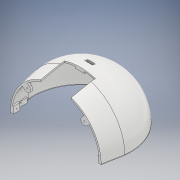
# Autodesk Inventor part: back
Saved by Autodesk Inventor 2017 (Build 210142000, 142)
## iProperties
Part Number: back
Material: Genérico
Document SubType Name: Modeling
Designer: Roberto
Density: 1 g/cm^3
Appearance: Valor por defecto
Author: Roberto
Autodesk Inventor part; units mm, degrees
ref_plane "YZ Plane" through (0, 0, 0) normal (1, 0, 0) x (0, 1, 0)
ref_plane "XY Plane" through (0, 0, 0) normal (0, 0, 1) x (1, 0, 0)
sketch "Boceto1" plane through (0, 0, 0) normal (0, 0, 1) x (1, 0, 0)
  line L0 (0, 0) -> (0.3056, 0)
  line L1 (-0.374, 3.3479) -> (0.2767, 0)
  line L2 (-0.6113, 3.2908) -> (0, 0)
  arc A0 (3.9618, 11.347) -> (-0.374, 3.3479) centre (7.6858, 4.1538) ccw
  arc A1 (3.8504, 11.5616) -> (-0.6113, 3.2908) centre (7.6858, 4.1538) ccw
  line L3 (0, 0) -> (15, 0)
  arc A2 (7.5, 12.385) -> (3.8946, 11.3118) centre (8.3964, 2.7813) ccw
  arc A3 (7.5, 12.6279) -> (3.8504, 11.5616) centre (8.3964, 2.7813) ccw
  line L4 (0, 0) -> (0.3056, 0)
  line L5 (0.2767, 0) -> (-0.374, 3.3479)
  line L6 (-0.6113, 3.2908) -> (0, 0)
  line L7 (-0.6113, 3.2908) -> (-0.374, 3.3479)
  line L8 (0.2767, 0) -> (0, 0)
  line L9 (7.5, 12.6279) -> (7.5, 12.385)
  dimension "d0" = 15
  constraints: 20 end point, 11 point on circle, 4 centre point, 3 collinear, 3 horizontal, 2 coincident, 1 vertical
  measures "d0" distance of L0.start L3.end
revolve "Revolución1" add sketch "Boceto1" angle 180 about axis through (7.5, 12.6279, 0) along (0, 1, 0)
sketch "Boceto2" plane through (7.5, 0, 0) normal (0, -1, 0) x (1, 0, 0)
  circle A0 centre (4.734, 4.734) radius 0.1
  circle A1 centre (-4.734, 4.734) radius 0.1
  arc A2 (7.5, 0) -> (-7.5, 0) centre (0, 0) ccw projected
  arc A3 (-5.1946, 4.3495) -> (-4.3495, 5.1946) centre (-4.734, 4.734) ccw
  line L0 (-4.2734, 5.1185) -> (-4.7635, 5.6086)
  line L1 (-5.1185, 4.2734) -> (-5.6117, 4.7666)
  line L2 (0, 0) -> (0, 11.2939)
  circle A4 centre (4.734, 4.734) radius 0.1
  arc A5 (7.5, 0) -> (-7.5, 0) centre (0, 0) ccw
  arc A6 (4.3495, 5.1946) -> (5.1946, 4.3495) centre (4.734, 4.734) ccw
  line L3 (4.2734, 5.1185) -> (4.8639, 5.709)
  line L4 (5.1185, 4.2734) -> (5.6108, 4.7657)
  line L5 (-4.6631, 5.5082) -> (-4.7635, 5.6086)
  line L6 (-5.5144, 4.6693) -> (-5.6117, 4.7666)
  line L7 (-5.6117, 4.7666) -> (-4.7635, 5.6086)
  arc A7 (7.2233, 0) -> (-7.2233, 0) centre (0, 0) ccw projected
  line L8 (5.5127, 4.6675) -> (5.6108, 4.7657)
  line L9 (4.6675, 5.5127) -> (4.7657, 5.6108)
  line L10 (4.7657, 5.6108) -> (5.6108, 4.7657)
  point P0 (-4.8639, 5.709)
  point P1 (-5.709, 4.8639)
  point P2 (5.709, 4.8639)
  dimension "d2" = 1.2
  dimension "d109" = 0.2
  dimension "d110" = 0.2
  constraints: 22 end point, 12 point on circle, 10 symmetric about line, 8 point on line, 6 centre point, 2 coincident, 2 parallel, 1 collinear, 1 vertical, 3 other
  measures "d2" diameter of A3
  measures "d109" diameter of A0
  measures "d110" diameter of A1
extrude "Extrusión1" add sketch "Boceto2" against normal blind 0.3 contours L10 L4 A7 L3 | A7 L4 A6 L3 | L1 A7 L0 A3 | L1 L7 L0 A7
sketch "Boceto4" plane through (7.6858, 4.1538, 0) normal (0, 0, -1) x (-0.8801071, 0.4747751, 0)
  line L0 (2.2994, -5.96) -> (-5.9165, -1.5279) projected
  line L1 (-4.0528, -2.5333) -> (-2.1537, 0.9871)
  line L2 (-2.1537, 0.9871) -> (2.3348, -1.4342)
  line L3 (2.3348, -1.4342) -> (0.4357, -4.9546)
  line L4 (-4.0528, -2.5333) -> (0.4357, -4.9546)
  line L5 (4.7922, -7.3048) -> (-8.4094, -0.1832) projected
  dimension "d6" = 4
  dimension "d7" = 5.1
  constraints: 8 end point, 2 point on line, 1 collinear, 1 perpendicular
  measures "d6" distance of L1.start L1.end
  measures "d7" distance of L1.end L2.end
extrude "Extrusión2" cut sketch "Boceto4" against normal blind 10
sketch "Boceto5" plane through (7.6858, 4.1538, 0) normal (0, 0, -1) x (-0.8801071, 0.4747751, 0)
  line L0 (-7.385, 3.0033) -> (-8.4094, -0.1832) projected
  line L1 (-8.4094, -0.1832) -> (-8.1658, -0.3145) projected
  line L2 (-8.1658, -0.3145) -> (-7.149, 2.941) projected
  arc A0 (0.3888, 7.9233) -> (-7.149, 2.941) centre (0.3271, -0.1764) ccw projected
  arc A1 (4.0715, 7.1562) -> (0.3888, 7.9233) centre (0.3008, -1.7218) ccw projected
  arc A2 (6.7351, 4.4998) -> (4.0715, 7.1562) centre (-1.277, -0.8706) ccw projected
  arc A3 (6.7109, -4.5358) -> (6.7351, 4.4998) centre (0, 0) ccw projected
  line L3 (4.5487, -7.1734) -> (6.7109, -4.5358) projected
  line L4 (4.7922, -7.3048) -> (4.5487, -7.1734) projected
  line L5 (6.8926, -4.6988) -> (4.7922, -7.3048) projected
  arc A4 (6.8926, -4.6988) -> (6.8926, 4.6988) centre (0, 0) ccw projected
  arc A5 (6.8926, 4.6988) -> (4.1869, 7.37) centre (-1.277, -0.8706) ccw projected
  arc A6 (4.1869, 7.37) -> (0.4686, 8.1642) centre (0.3008, -1.7218) ccw projected
  arc A7 (0.4686, 8.1642) -> (-7.385, 3.0033) centre (0.3271, -0.1764) ccw projected
extrude "Extrusión3" add sketch "Boceto5" along normal blind 0.1
sketch "Boceto6" plane through (7.5, 4, 0) normal (0, -1, 0) x (1, 0, 0)
  arc A0 (2.55, 7.7457) -> (-2.55, 7.7457) centre (0, 0) ccw projected
  line L0 (-2.55, 7.4906) -> (-2.55, 7.7457) projected
  arc A1 (2.55, 7.4906) -> (-2.55, 7.4906) centre (0, 0) ccw projected
  line L1 (2.55, 7.4906) -> (2.55, 7.7457) projected
  arc A2 (2.55, 7.7457) -> (-2.55, 7.7457) centre (0, 0) ccw projected
  line L2 (0, 8.1546) -> (0, 7.9127)
  line L3 (0, 8.0337) -> (-0.75, 8.0337)
  line L4 (-0.75, 8.0337) -> (-0.75, 7.5837)
  line L5 (-0.75, 7.5837) -> (0.75, 7.5837)
  line L6 (0.75, 7.5837) -> (0.75, 8.0337)
  line L7 (0.75, 8.0337) -> (0, 8.0337)
  point P0 (-7.5, 0)
  dimension "d12" = 0.75
  dimension "d13" = 0.45
  dimension "d14" = 1.5
  constraints: 12 end point, 4 perpendicular, 3 point on circle, 1 horizontal, 1 midpoint, 1 point on line
  measures "d12" distance of L3.start L3.end
  measures "d13" distance of L3.end L4.end
  measures "d14" distance of L4.end L5.end
extrude "Extrusión4" add sketch "Boceto6" against normal blind 1.2 contours L7 L6 A1 L2 | L2 A1 L4 L3 | L6 L5 L4 A1
sketch "Boceto7" plane through (8.25, 4, 7.5837) normal (0, 0, -1) x (-1, 0, 0)
  line L0 (1.5, 0) -> (0, 0) projected
  line L1 (1.5, 0) -> (1.5, 1.2) projected
  line L2 (0, 1.2) -> (1.5, 1.2) projected
  line L3 (0, 0) -> (0, 1.2) projected
  line L4 (0, 1.2) -> (1.5, 1.2) projected
  line L5 (3.3, 0) -> (-1.8, 0) projected
  circle A0 centre (0.65, 0.3) radius 0.075
  circle A1 centre (0.65, 0.9) radius 0.075
  point P0 (8.25, -4)
  dimension "d20" = 0.15
  dimension "d21" = 0.15
  constraints: 2 centre point
  measures "d20" diameter of A0
  measures "d21" diameter of A1
extrude "Extrusión5" cut sketch "Boceto7" against normal blind 0.3 contours A0 | A1
ref_plane "Plano de trabajo1" through (0, 2, 0) normal (0, 1, 0) x (-1, 0, 0)
sketch "Boceto12" plane through (0, 2, 0) normal (0, 1, 0) x (-1, 0, 0)
  line L0 (-15, -0.1) -> (-15.6113, -0.1)
  line L1 (-0.3817, -3.084) -> (-1.27, -4.6226)
  line L2 (-1.27, -4.6226) -> (-1.4865, -4.4976)
  line L3 (-4.541, -6.9018) -> (-3.0024, -6.0135)
  line L4 (-2.8774, -6.23) -> (-3.0024, -6.0135)
  line L5 (-0.3817, -3.084) -> (-0.5982, -2.959)
  line L6 (-6.6117, -7.7066) -> (-8.3883, -7.7066)
  line L7 (-8.3883, -7.7066) -> (-8.3883, -7.4566)
  line L8 (-1.4865, -4.4976) -> (-0.5982, -2.959)
  line L9 (-2.8774, -6.23) -> (-4.416, -7.1183)
  line L10 (-4.416, -7.1183) -> (-4.541, -6.9018)
  line L11 (-8.3883, -7.4566) -> (-6.6117, -7.4566)
  line L12 (-6.6117, -7.7066) -> (-6.6117, -7.4566)
  line L13 (-0.0434, -0.1) -> (0.2066, -0.1)
  line L14 (-7.5, 0) -> (-7.5, -4.1757)
  line L15 (-14.6183, -3.084) -> (-13.73, -4.6226)
  line L16 (-13.73, -4.6226) -> (-13.5135, -4.4976)
  line L17 (-15.2066, -1.0883) -> (-14.9566, -1.0883)
  line L18 (-13.5135, -4.4976) -> (-14.4018, -2.959)
  line L19 (-14.6183, -3.084) -> (-14.4018, -2.959)
  line L20 (-15.2066, -1.0883) -> (-14.9566, -1.0883)
  line L21 (-14.9566, -1.0883) -> (-14.9566, -0.1)
  line L22 (-15.2066, -0.1) -> (-15.2066, -1.0883)
  line L23 (-14.7233, -0.1) -> (-15.374, -0.1)
  line L24 (-14.9566, -0.1) -> (-15.2066, -0.1)
  line L25 (-10.459, -6.9018) -> (-11.9976, -6.0135)
  line L26 (-12.1226, -6.23) -> (-11.9976, -6.0135)
  line L27 (-12.1226, -6.23) -> (-10.584, -7.1183)
  line L28 (-10.584, -7.1183) -> (-10.459, -6.9018)
  line L29 (-6.6117, -7.7066) -> (-8.3883, -7.7066)
  line L30 (-8.3883, -7.7066) -> (-8.3883, -7.4566)
  line L31 (-8.3883, -7.4566) -> (-6.6117, -7.4566)
  line L32 (-6.6117, -7.4566) -> (-6.6117, -7.7066)
  line L33 (-2.8774, -6.23) -> (-3.0024, -6.0135)
  line L34 (-2.8774, -6.23) -> (-4.416, -7.1183)
  line L35 (-4.416, -7.1183) -> (-4.541, -6.9018)
  line L36 (-4.541, -6.9018) -> (-3.0024, -6.0135)
  line L37 (-10.584, -7.1183) -> (-12.1226, -6.23)
  line L38 (-12.1226, -6.23) -> (-11.9976, -6.0135)
  line L39 (-11.9976, -6.0135) -> (-10.459, -6.9018)
  line L40 (-10.459, -6.9018) -> (-10.584, -7.1183)
  line L41 (-13.5135, -4.4976) -> (-13.73, -4.6226)
  line L42 (-13.73, -4.6226) -> (-14.6183, -3.084)
  line L43 (-14.6183, -3.084) -> (-14.4018, -2.959)
  line L44 (-14.4018, -2.959) -> (-13.5135, -4.4976)
  line L45 (-15.2066, -0.1) -> (-14.9566, -0.1)
  line L46 (-14.9566, -0.1) -> (-14.9566, -1.0883)
  line L47 (-14.9566, -1.0883) -> (-15.2066, -1.0883)
  line L48 (-15.2066, -1.0883) -> (-15.2066, -0.1)
  line L49 (-2.8774, -6.23) -> (-3.0024, -6.0135)
  line L50 (-4.416, -7.1183) -> (-2.8774, -6.23)
  line L51 (-3.0024, -6.0135) -> (-4.541, -6.9018)
  line L52 (-4.541, -6.9018) -> (-4.416, -7.1183)
  line L53 (-0.3817, -3.084) -> (-0.5982, -2.959)
  line L54 (-0.5982, -2.959) -> (-1.4865, -4.4976)
  line L55 (-1.4865, -4.4976) -> (-1.27, -4.6226)
  line L56 (-1.27, -4.6226) -> (-0.3817, -3.084)
  line L57 (0.2066, -0.1) -> (-0.0434, -0.1)
  line L58 (0.374, -0.1) -> (0.4955, -0.2591)
  line L59 (-0.0434, 0.6887) -> (0.2066, 0.6887)
  line L60 (0.2066, 0.6887) -> (0.2066, -0.1)
  line L61 (0.2066, -0.1) -> (-0.0434, -0.1)
  line L62 (-0.0434, 0.6887) -> (-0.0434, -0.1)
  line L63 (0.2066, -0.1) -> (-0.0434, -0.1)
  line L64 (-15.2066, -0.1) -> (-14.9566, -0.1)
  line L65 (-14.9566, -0.1) -> (-15.2066, -0.1)
  line L66 (-15.2066, 0.6887) -> (-14.9566, 0.6887)
  line L67 (-14.9566, 0.6887) -> (-14.9566, -0.1)
  line L68 (-14.9566, -0.1) -> (-15.2066, -0.1)
  line L69 (-15.2066, 0.6887) -> (-15.2066, -0.1)
  line L70 (-14.9566, -0.1) -> (-15.2066, -0.1)
  point P0 (0, 0)
  point P1 (0, -0.2)
  point P2 (-15, -0.2)
  point P3 (-15.1632, -0.2)
  dimension "d34" = 0.25
  dimension "d36" = 0.25
  dimension "d37" = 0.25
  dimension "d39" = 0.25
  dimension "d40" = 0.25
  constraints: 142 end point, 18 perpendicular, 13 symmetric about line, 6 parallel, 5 collinear, 3 horizontal, 3 vertical, 1 point on line
  measures "d34" distance of L2.end L1.end
  measures "d36" distance of L31.start L6.end
  measures "d37" distance of L10.start L10.end
  measures "d39" distance of L59.start L59.end
  measures "d40" distance of L66.start L66.end
extrude "Extrusión8" add sketch "Boceto12" along normal blind 0.735 and the other way blind 0.535 contours L0 L69 L66 L67 L23 | L62 L59 L60 L13
sketch "Boceto13" plane through (0.0434, 1.465, -0.1) normal (1, 0, 0) x (0, 0, -1)
  line L0 (-0.473, 0.6898) -> (-0.613, 0.6898)
  circle A0 centre (0.3713, 1.15) radius 0.06
  line L1 (-0.0207, 0.3598) -> (-0.0207, 0.8098)
  line L2 (0.2193, 0.8098) -> (0.2193, 0.3598)
  line L3 (-0.7887, 1.27) -> (0.9913, 1.27)
  line L4 (0.9913, 0) -> (-0.7887, 0)
  line L5 (0.9913, 1.27) -> (0.003, 1.27)
  circle A1 centre (0.7413, 0.25) radius 0.11
  line L6 (0.9913, 1.27) -> (0.9913, 0)
  circle A2 centre (0.8713, 1.15) radius 0.06
  circle A3 centre (0.6113, 1.15) radius 0.06
  line L7 (-0.0207, 0.8098) -> (0.2193, 0.8098)
  circle A4 centre (0.1113, 1.15) radius 0.06
  circle A5 centre (-0.1487, 1.15) radius 0.06
  circle A6 centre (-0.4087, 1.15) radius 0.06
  line L8 (-0.473, 0.9898) -> (-0.473, 0.6898)
  circle A7 centre (-0.6687, 1.15) radius 0.06
  line L9 (-0.613, 0.9898) -> (-0.473, 0.9898)
  line L10 (-0.613, 0.6898) -> (-0.613, 0.9898)
  line L11 (0.2193, 0.3598) -> (-0.0207, 0.3598)
  circle A8 centre (-0.5387, 0.25) radius 0.11
  line L12 (-0.7887, 0) -> (0.003, 0)
  line L13 (-0.7887, 0) -> (-0.7887, 0.25)
  line L14 (0.003, 1.27) -> (0.003, 0)
  line L15 (0.003, 0) -> (0.003, 1.27)
  line L16 (-0.7887, 1.27) -> (-0.7887, 0)
  line L17 (-0.7887, 1.27) -> (-0.7887, 1.15)
  line L18 (-0.7887, 1.27) -> (-0.7887, 0)
  line L19 (0.003, 1.27) -> (-0.7887, 1.27)
  line L20 (-0.473, 0.6898) -> (-0.613, 0.6898)
  circle A9 centre (0.3713, 1.15) radius 0.06
  line L21 (-0.0207, 0.3598) -> (-0.0207, 0.8098)
  line L22 (0.2193, 0.8098) -> (0.2193, 0.3598)
  line L23 (-0.7887, 1.27) -> (0.9913, 1.27)
  line L24 (0.9913, 0) -> (-0.7887, 0)
  line L25 (0.9913, 1.27) -> (0.003, 1.27)
  circle A10 centre (0.7413, 0.25) radius 0.11
  line L26 (0.9913, 1.27) -> (0.9913, 0)
  circle A11 centre (0.8713, 1.15) radius 0.06
  circle A12 centre (0.6113, 1.15) radius 0.06
  line L27 (-0.0207, 0.8098) -> (0.2193, 0.8098)
  circle A13 centre (0.1113, 1.15) radius 0.06
  circle A14 centre (-0.1487, 1.15) radius 0.06
  circle A15 centre (-0.4087, 1.15) radius 0.06
  line L28 (-0.473, 0.9898) -> (-0.473, 0.6898)
  circle A16 centre (-0.6687, 1.15) radius 0.06
  line L29 (-0.613, 0.9898) -> (-0.473, 0.9898)
  line L30 (-0.613, 0.6898) -> (-0.613, 0.9898)
  line L31 (0.2193, 0.3598) -> (-0.0207, 0.3598)
  circle A17 centre (-0.5387, 0.25) radius 0.11
  line L32 (-0.7887, 0) -> (0.003, 0)
  line L33 (-0.7887, 0) -> (-0.7887, 0.25)
  line L34 (0.003, 1.27) -> (0.003, 0)
  line L35 (0.003, 0) -> (0.003, 1.27)
  line L36 (-0.7887, 1.27) -> (-0.7887, 0)
  line L37 (-0.7887, 1.27) -> (-0.7887, 1.15)
  line L38 (-0.7887, 1.27) -> (-0.7887, 0)
  line L39 (0.003, 1.27) -> (-0.7887, 1.27)
  line L40 (-0.473, 0.6898) -> (-0.613, 0.6898)
  circle A18 centre (0.3713, 1.15) radius 0.06
  line L41 (-0.0207, 0.3598) -> (-0.0207, 0.8098)
  line L42 (0.2193, 0.8098) -> (0.2193, 0.3598)
  line L43 (-0.7887, 1.27) -> (0.9913, 1.27)
  line L44 (0.9913, 0) -> (-0.7887, 0)
  line L45 (0.9913, 1.27) -> (0.003, 1.27)
  circle A19 centre (0.7413, 0.25) radius 0.11
  line L46 (0.9913, 1.27) -> (0.9913, 0)
  circle A20 centre (0.8713, 1.15) radius 0.06
  circle A21 centre (0.6113, 1.15) radius 0.06
  line L47 (-0.0207, 0.8098) -> (0.2193, 0.8098)
  circle A22 centre (0.1113, 1.15) radius 0.06
  circle A23 centre (-0.1487, 1.15) radius 0.06
  circle A24 centre (-0.4087, 1.15) radius 0.06
  line L48 (-0.473, 0.9898) -> (-0.473, 0.6898)
  circle A25 centre (-0.6687, 1.15) radius 0.06
  line L49 (-0.613, 0.9898) -> (-0.473, 0.9898)
  line L50 (-0.613, 0.6898) -> (-0.613, 0.9898)
  line L51 (0.2193, 0.3598) -> (-0.0207, 0.3598)
  circle A26 centre (-0.5387, 0.25) radius 0.11
  line L52 (-0.7887, 0) -> (0.003, 0)
  line L53 (-0.7887, 0) -> (-0.7887, 0.25)
  line L54 (0.003, 1.27) -> (0.003, 0)
  line L55 (0.003, 0) -> (0.003, 1.27)
  line L56 (-0.7887, 1.27) -> (-0.7887, 0)
  line L57 (-0.7887, 1.27) -> (-0.7887, 1.15)
  line L58 (-0.7887, 1.27) -> (-0.7887, 0)
  line L59 (0.003, 1.27) -> (-0.7887, 1.27)
  point P0 (-0.1, -1.465)
  point P1 (0.9913, 1.27)
  point P2 (0.9913, 1.27)
  point P3 (0.9913, 1.27)
  point P4 (0.9913, 1.27)
  point P5 (0.9913, 1.27)
  point P6 (0.9913, 1.27)
  point P7 (-0.7887, 1.27)
  constraints: 120 end point, 27 centre point, 9 point on line
extrude "Extrusión9" cut sketch "Boceto13" against normal blind 0.723 contours L1 L7 L14 L11 | L14 L7 L2 L11
sketch "Boceto14" plane through (0.0434, 1.465, 0.6887) normal (1, 0, 0) x (0, 0, -1)
  line L0 (0.1993, 0.7544) -> (0.2948, 0.7544)
  circle A0 centre (0.1614, 0.8636) radius 0.0409
  line L1 (0.0795, 0.9455) -> (0.0795, 0.8636)
  line L2 (0.6193, 0.9455) -> (0.0795, 0.9455)
  circle A1 centre (0.3386, 0.8636) radius 0.0409
  circle A2 centre (0.5159, 0.8636) radius 0.0409
  line L3 (0.2948, 0.5499) -> (0.1993, 0.5499)
  line L4 (0.2948, 0.7544) -> (0.2948, 0.5499)
  line L5 (0.1993, 0.5499) -> (0.1993, 0.7544)
  line L6 (0.6032, 0.6317) -> (0.7668, 0.6317)
  line L7 (0.0795, 0.9455) -> (0.0795, 0.0795)
  line L8 (0.0795, 0.9455) -> (0.0795, 0.0795)
  line L9 (0.6193, 0.9455) -> (0.6193, 0.0795)
  line L10 (0.6193, 0.0795) -> (0.6193, 0.9455)
  line L11 (0.6032, 0.3248) -> (0.6032, 0.6317)
  line L12 (0.7668, 0.6317) -> (0.7668, 0.3248)
  line L13 (0.7668, 0.3248) -> (0.6032, 0.3248)
  line L14 (0.0795, 0.0795) -> (0.6193, 0.0795)
  line L15 (0.0795, 0.0795) -> (0.0795, 0.25)
  circle A3 centre (0.25, 0.25) radius 0.075
  circle A4 centre (0.8705, 0.8636) radius 0.0409
  line L16 (0.0795, 0.9455) -> (1.2932, 0.9455)
  line L17 (1.2932, 0.0795) -> (0.0795, 0.0795)
  line L18 (1.2932, 0.9455) -> (0.6193, 0.9455)
  circle A5 centre (1.1227, 0.25) radius 0.075
  line L19 (1.2932, 0.9455) -> (1.2932, 0.0795)
  circle A6 centre (0.6932, 0.8636) radius 0.0409
  circle A7 centre (1.0341, 0.8636) radius 0.0409
  circle A8 centre (1.2114, 0.8636) radius 0.0409
  line L20 (0.1993, 0.7544) -> (0.2948, 0.7544)
  circle A9 centre (0.1614, 0.8636) radius 0.0409
  line L21 (0.0795, 0.9455) -> (0.0795, 0.8636)
  line L22 (0.6193, 0.9455) -> (0.0795, 0.9455)
  circle A10 centre (0.3386, 0.8636) radius 0.0409
  circle A11 centre (0.5159, 0.8636) radius 0.0409
  line L23 (0.2948, 0.5499) -> (0.1993, 0.5499)
  line L24 (0.2948, 0.7544) -> (0.2948, 0.5499)
  line L25 (0.1993, 0.5499) -> (0.1993, 0.7544)
  line L26 (0.6032, 0.6317) -> (0.7668, 0.6317)
  line L27 (0.0795, 0.9455) -> (0.0795, 0.0795)
  line L28 (0.0795, 0.9455) -> (0.0795, 0.0795)
  line L29 (0.6193, 0.9455) -> (0.6193, 0.0795)
  line L30 (0.6193, 0.0795) -> (0.6193, 0.9455)
  line L31 (0.6032, 0.3248) -> (0.6032, 0.6317)
  line L32 (0.7668, 0.6317) -> (0.7668, 0.3248)
  line L33 (0.7668, 0.3248) -> (0.6032, 0.3248)
  line L34 (0.0795, 0.0795) -> (0.6193, 0.0795)
  line L35 (0.0795, 0.0795) -> (0.0795, 0.25)
  circle A12 centre (0.25, 0.25) radius 0.075
  circle A13 centre (0.8705, 0.8636) radius 0.0409
  line L36 (0.0795, 0.9455) -> (1.2932, 0.9455)
  line L37 (1.2932, 0.0795) -> (0.0795, 0.0795)
  line L38 (1.2932, 0.9455) -> (0.6193, 0.9455)
  circle A14 centre (1.1227, 0.25) radius 0.075
  line L39 (1.2932, 0.9455) -> (1.2932, 0.0795)
  circle A15 centre (0.6932, 0.8636) radius 0.0409
  circle A16 centre (1.0341, 0.8636) radius 0.0409
  circle A17 centre (1.2114, 0.8636) radius 0.0409
  line L40 (0.1993, 0.7544) -> (0.2948, 0.7544)
  circle A18 centre (0.1614, 0.8636) radius 0.0409
  line L41 (0.0795, 0.9455) -> (0.0795, 0.8636)
  line L42 (0.6193, 0.9455) -> (0.0795, 0.9455)
  circle A19 centre (0.3386, 0.8636) radius 0.0409
  circle A20 centre (0.5159, 0.8636) radius 0.0409
  line L43 (0.2948, 0.5499) -> (0.1993, 0.5499)
  line L44 (0.2948, 0.7544) -> (0.2948, 0.5499)
  line L45 (0.1993, 0.5499) -> (0.1993, 0.7544)
  line L46 (0.6032, 0.6317) -> (0.7668, 0.6317)
  line L47 (0.0795, 0.9455) -> (0.0795, 0.0795)
  line L48 (0.0795, 0.9455) -> (0.0795, 0.0795)
  line L49 (0.6193, 0.9455) -> (0.6193, 0.0795)
  line L50 (0.6193, 0.0795) -> (0.6193, 0.9455)
  line L51 (0.6032, 0.3248) -> (0.6032, 0.6317)
  line L52 (0.7668, 0.6317) -> (0.7668, 0.3248)
  line L53 (0.7668, 0.3248) -> (0.6032, 0.3248)
  line L54 (0.0795, 0.0795) -> (0.6193, 0.0795)
  line L55 (0.0795, 0.0795) -> (0.0795, 0.25)
  circle A21 centre (0.25, 0.25) radius 0.075
  circle A22 centre (0.8705, 0.8636) radius 0.0409
  line L56 (0.0795, 0.9455) -> (1.2932, 0.9455)
  line L57 (1.2932, 0.0795) -> (0.0795, 0.0795)
  line L58 (1.2932, 0.9455) -> (0.6193, 0.9455)
  circle A23 centre (1.1227, 0.25) radius 0.075
  line L59 (1.2932, 0.9455) -> (1.2932, 0.0795)
  circle A24 centre (0.6932, 0.8636) radius 0.0409
  circle A25 centre (1.0341, 0.8636) radius 0.0409
  circle A26 centre (1.2114, 0.8636) radius 0.0409
  point P0 (0.6887, -1.465)
  point P1 (1.2932, 0.9455)
  point P2 (1.2932, 0.9455)
  point P3 (1.2932, 0.9455)
  point P4 (1.2932, 0.9455)
  point P5 (1.2932, 0.9455)
  point P6 (1.2932, 0.9455)
  point P7 (0.0795, 0.9455)
  point P8 (0, 1.27)
  dimension "d111" = 0.15
  constraints: 120 end point, 27 centre point, 9 point on line
  measures "d111" diameter of A21
extrude "Extrusión10" cut sketch "Boceto14" against normal blind 0.15 contours A3
sketch "Boceto15" plane through (14.9566, 1.465, 0.6887) normal (-1, 0, 0) x (0, 0, 1)
  circle A0 centre (-0.25, 0.25) radius 0.075 projected
  circle A1 centre (-0.25, 0.25) radius 0.075 projected
  line L0 (-0.7887, 0.3598) -> (-0.768, 0.3598) projected
  line L1 (-0.768, 0.3598) -> (-0.768, 0.8098) projected
  line L2 (-0.768, 0.8098) -> (-0.7887, 0.8098) projected
  line L3 (-0.7887, 1.27) -> (-0.7887, 0.8098) projected
  line L4 (0, 1.27) -> (-0.7887, 1.27) projected
  line L5 (0, 0) -> (0, 1.27) projected
  line L6 (-0.7887, 0) -> (0, 0) projected
  line L7 (-0.7887, 0.3598) -> (-0.7887, 0) projected
  line L8 (-0.7887, 0.8098) -> (-0.768, 0.8098)
  line L9 (-0.768, 0.8098) -> (-0.768, 0.3598)
  line L10 (-0.768, 0.3598) -> (-0.7887, 0.3598)
  line L11 (-0.7887, 0.3598) -> (-0.7887, 0.8098)
  point P0 (-0.6887, -1.465)
  constraints: 8 end point, 2 parallel, 1 horizontal, 1 perpendicular
extrude "Extrusión11" cut sketch "Boceto15" against normal blind 15 contours L11 L2 L1 L0
sketch "Boceto16" plane through (14.9566, 1.465, 0.6887) normal (-1, 0, 0) x (0, 0, 1)
  circle A0 centre (-0.25, 0.25) radius 0.11
  line L0 (-0.7887, 0.3598) -> (-0.768, 0.3598)
  line L1 (-0.768, 0.3598) -> (-0.768, 0.8098)
  line L2 (-0.768, 0.8098) -> (-0.7887, 0.8098)
  line L3 (-0.7887, 1.27) -> (-0.7887, 0.8098)
  line L4 (0, 1.27) -> (-0.7887, 1.27)
  line L5 (0, 0) -> (0, 1.27)
  line L6 (-0.7887, 0) -> (0, 0)
  line L7 (-0.7887, 0.3598) -> (-0.7887, 0)
  line L8 (-0.7887, 0.8098) -> (-0.768, 0.8098)
  line L9 (-0.768, 0.8098) -> (-0.768, 0.3598)
  line L10 (-0.768, 0.3598) -> (-0.7887, 0.3598)
  line L11 (-0.7887, 0.3598) -> (-0.7887, 0.8098)
  circle A1 centre (-0.25, 0.25) radius 0.075
  point P0 (-0.6887, -1.465)
  dimension "d113" = 0.15
  constraints: 24 end point, 2 centre point, 2 parallel, 1 coincident, 1 horizontal, 1 perpendicular
  measures "d113" diameter of A1
extrude "Extrusión12" cut sketch "Boceto16" against normal blind 0.15 contours A1
sketch "Boceto17" plane through (7.6858, 4.1538, -0.1) normal (0, 0, -1) x (-0.8801071, 0.4747751, 0)
  arc A0 (6.7351, 4.4998) -> (4.0715, 7.1562) centre (-1.277, -0.8706) ccw projected
  arc A1 (4.0715, 7.1562) -> (0.3888, 7.9233) centre (0.3008, -1.7218) ccw projected
  line L0 (6.7351, 4.4998) -> (0.3888, 7.9233) projected
  line L1 (4.0715, 7.1562) -> (3.562, 6.2116)
  line L2 (6.7351, 4.4998) -> (0.3888, 7.9233) projected
  line L3 (3.562, 6.2116) -> (0.3888, 7.9233)
  arc A2 (4.0715, 7.1562) -> (0.3888, 7.9233) centre (0.3008, -1.7218) ccw
  point P0 (4.7922, -7.3048)
  constraints: 4 end point, 2 point on circle, 1 centre point, 1 collinear, 1 concentric, 1 midpoint
revolve "Revolución2" add sketch "Boceto17" angle 180 about axis through (7.5, 12.385, -0.1) along (0, -1, 0) contours L1 L0 A1
sketch "Boceto18" plane through (11.1054, 11.3118, -0.1) normal (0, 0, -1) x (-1, 0, 0)
  arc A0 (3.6054, 1.0733) -> (0, 0) centre (4.5018, -8.5305) ccw
  line L0 (0, 0) -> (7.2108, 0)
  arc A1 (7.2108, 0) -> (3.6054, 1.0733) centre (2.709, -8.5305) ccw
  arc A2 (7.2108, 0) -> (3.6054, 1.0733) centre (2.709, -8.5305) ccw
  line L1 (7.2108, 0) -> (3.6054, 0)
  line L2 (0, 0) -> (7.2108, 0)
  line L3 (3.6054, 0.1866) -> (4.4054, 0.1866)
  line L4 (4.4054, 0.1866) -> (4.4054, 0.7866)
  line L5 (4.4054, 0.7866) -> (2.8054, 0.7866)
  line L6 (2.8054, 0.7866) -> (2.8054, 0.1866)
  line L7 (2.8054, 0.1866) -> (3.6054, 0.1866)
  arc A3 (3.6054, 1.0733) -> (0, 0) centre (4.5018, -8.5305) ccw
  line L8 (0, 0) -> (7.2108, 0)
  arc A4 (7.2108, 0) -> (3.6054, 1.0733) centre (2.709, -8.5305) ccw
  arc A5 (7.2108, 0) -> (3.6054, 1.0733) centre (2.709, -8.5305) ccw
  line L9 (7.2108, 0) -> (3.6054, 0)
  line L10 (0, 0) -> (7.2108, 0)
  line L11 (3.6054, 0.1866) -> (4.4054, 0.1866)
  line L12 (4.4054, 0.1866) -> (4.4054, 0.7866)
  line L13 (4.4054, 0.7866) -> (2.8054, 0.7866)
  line L14 (2.8054, 0.7866) -> (2.8054, 0.1866)
  line L15 (2.8054, 0.1866) -> (3.6054, 0.1866)
  line L16 (2.8354, 0.7566) -> (4.3754, 0.7566)
  line L17 (4.3754, 0.7566) -> (4.3754, 0.2166)
  line L18 (4.3754, 0.2166) -> (3.6054, 0.2166)
  line L19 (3.6054, 0.2166) -> (2.8354, 0.2166)
  line L20 (2.8354, 0.2166) -> (2.8354, 0.7566)
  point P0 (11.1054, -11.3118)
  dimension "d54" = 0.8
  dimension "d55" = 0.6
  dimension "d56" = 1.6
  dimension "d57" = 0.6
  dimension "d58" = 0.8
  dimension "d59" = 0.6
  dimension "d60" = 1.6
  dimension "d61" = 0.6
  dimension "d62" = 0.03
  constraints: 42 end point, 12 point on circle, 6 centre point, 6 perpendicular, 3 collinear, 2 midpoint, 2 point on line, 4 other
  measures "d54" distance of L3.start L3.end
  measures "d55" distance of L3.end L4.end
  measures "d56" distance of L4.end L5.end
  measures "d57" distance of L5.end L6.end
  measures "d58" distance of L11.start L11.end
  measures "d59" distance of L11.end L12.end
  measures "d60" distance of L12.end L13.end
  measures "d61" distance of L13.end L14.end
  measures "d62" distance between parallel lines of L5 L16
extrude "Extrusión13" add sketch "Boceto18" along normal blind 0.32 contours L16 L17 L18 L19 L20
sketch "Boceto19" plane through (7.5, 11.3118, -0.1) normal (0, -1, 0) x (1, 0, 0)
  line L0 (3.6054, 0) -> (-3.6054, 0) projected
  arc A0 (3.6054, 0) -> (-3.6054, 0) centre (0, 0) ccw projected
  circle A1 centre (0, 0) radius 1.5
  line L1 (1.5, 0) -> (1.5, 0.8)
  circle A2 centre (1.5, 0.8) radius 0.15
  line L2 (-1.5, 0) -> (-1.5, 0.8)
  circle A3 centre (-1.5, 0.8) radius 0.15
  point P0 (-7.5, 0.1)
  dimension "d65" = 3
  dimension "d66" = 0.8
  dimension "d67" = 0.3
  dimension "d68" = 0.8
  dimension "d69" = 0.3
  constraints: 4 end point, 3 centre point, 3 coincident, 2 point on circle, 2 point on line, 2 tangent, 2 vertical
  measures "d65" diameter of A1
  measures "d66" distance of L1.start L1.end
  measures "d67" diameter of A2
  measures "d68" distance of L2.start L2.end
  measures "d69" diameter of A3
extrude "Extrusión14" cut sketch "Boceto19" against normal blind 0.35 contours A2 | A3
sketch "Boceto21" plane through (7.5, 5.2, 0) normal (0, 1, 0) x (1, 0, 0)
  arc A0 (-0.75, -7.8104) -> (0.75, -7.8104) centre (0, 0) ccw projected
  line L0 (0.75, -7.8104) -> (0.75, -7.5837) projected
  line L1 (0.75, -7.5837) -> (-0.75, -7.5837) projected
  line L2 (-0.75, -7.5837) -> (-0.75, -7.8104) projected
  point P0 (-7.5, 0)
extrude "Extrusión16" add sketch "Boceto21" along normal blind 1.1
sketch "Boceto22" plane through (8.25, 4, 7.5837) normal (0, 0, -1) x (-1, 0, 0)
  circle A0 centre (0.65, 0.3) radius 0.075 projected
  circle A1 centre (0.65, 0.9) radius 0.075 projected
  line L0 (1.5, 0) -> (0, 0) projected
  line L1 (1.5, 0) -> (1.5, 2.3) projected
  line L2 (0, 2.3) -> (1.5, 2.3) projected
  line L3 (0, 0) -> (0, 2.3) projected
  line L4 (0, 2.3) -> (1.5, 2.3) projected
  line L5 (0.75, 2.3) -> (0.75, 1.9)
  line L6 (0.75, 1.9) -> (0.125, 1.9)
  line L7 (0.125, 1.9) -> (0.125, 1.4)
  line L8 (0.125, 1.4) -> (1.375, 1.4)
  line L9 (1.375, 1.4) -> (1.375, 1.9)
  line L10 (1.375, 1.9) -> (0.75, 1.9)
  point P0 (8.25, -4)
  dimension "d83" = 0.4
  dimension "d84" = 0.625
  dimension "d85" = 0.5
  dimension "d86" = 1.25
  constraints: 12 end point, 4 perpendicular, 1 midpoint, 1 parallel, 1 point on line, 1 vertical
  measures "d83" distance of L5.start L5.end
  measures "d84" distance of L5.end L6.end
  measures "d85" distance of L6.end L7.end
  measures "d86" distance of L7.end L8.end
extrude "Extrusión17" cut sketch "Boceto22" against normal blind 1.1 contours L10 L9 L8 L7 L6
sketch "Boceto23" plane through (7.6858, 4.1538, -0.1) normal (0, 0, -1) x (-0.8801071, 0.4747751, 0)
  line L0 (5.4948, -6.0192) -> (4.5487, -7.1734) projected
  line L1 (4.5487, -7.1734) -> (3.0432, -6.3612) projected
  line L2 (5.4948, -6.0192) -> (5.4496, -5.9948) projected
  line L3 (4.8783, -6.1411) -> (4.3727, -7.0784)
  line L4 (4.5487, -7.1734) -> (4.3727, -7.0784)
  line L5 (-4.0528, -2.5333) -> (-5.9165, -1.5279) projected
  line L6 (-4.0528, -2.5333) -> (0.4588, -4.9671)
  line L7 (0.4588, -4.9671) -> (-1.797, -3.7502)
  line L8 (-3.1118, -6.1875) -> (-1.797, -3.7502)
  line L9 (-7.8424, 0.7211) -> (-8.1658, -0.3145)
  line L10 (-8.1658, -0.3145) -> (-6.6603, -1.1267)
  line L11 (-7.4841, 0.5278) -> (-7.9898, -0.4095)
  line L12 (-8.1658, -0.3145) -> (-7.9898, -0.4095)
  line L13 (5.2365, -6.3344) -> (4.5487, -7.1734)
  line L14 (4.5487, -7.1734) -> (4.3727, -7.0784)
  line L15 (4.3727, -7.0784) -> (4.8783, -6.1411)
  line L16 (-8.1658, -0.3145) -> (-7.7209, 1.11) projected
  line L17 (-7.4841, 0.5278) -> (-7.9898, -0.4095)
  line L18 (-6.6603, -1.1267) -> (-8.1658, -0.3145) projected
  line L19 (-7.9898, -0.4095) -> (-8.1658, -0.3145)
  line L20 (-8.1658, -0.3145) -> (-7.7209, 1.11) projected
  line L21 (-7.8424, 0.7211) -> (-8.1658, -0.3145)
  line L22 (4.8783, -6.1411) -> (5.2365, -6.3344)
  line L23 (-7.4841, 0.5278) -> (-7.8424, 0.7211)
  point P0 (4.7922, -7.3048)
  point P1 (-8.3863, -0.1956)
  constraints: 34 end point, 7 perpendicular, 3 collinear, 3 point on line, 1 midpoint, 1 symmetric about line
extrude "Extrusión18" add sketch "Boceto23" against normal blind 1.1
sketch "Boceto25" plane through (0.4767, 0, -0.1) normal (1, 0, 0) x (0, 0, -1)
  line L0 (0, 1.065) -> (0, 0) projected
  line L1 (0, 1.065) -> (-1.1, 1.065) projected
  line L2 (-1.1, 0) -> (-1.1, 1.065) projected
  line L3 (0, 0) -> (-1.1, 0) projected
  circle A0 centre (-0.5, 0.5325) radius 0.075
  point P0 (-0.1, 0)
  dimension "d95" = 0.15
  constraints: 1 centre point
  measures "d95" diameter of A0
extrude "Extrusión19" cut sketch "Boceto25" against normal blind 0.4 contours A0
sketch "Boceto26" plane through (14.5233, 0, -0.1) normal (-1, 0, 0) x (0, 0, 1)
  circle A0 centre (0.5, 0.5325) radius 0.075 projected
  point P0 (0.1, 0)
extrude "Extrusión20" cut sketch "Boceto26" against normal blind 0.4
sketch "Boceto27" plane through (11.1054, 11.3118, -0.1) normal (0, 0, -1) x (-1, 0, 0)
  line L0 (0, 0) -> (7.2108, 0) projected
  line L1 (0, 0) -> (-2.6819, 0)
  line L2 (-2.6819, 0) -> (-2.6819, 2.3953)
  line L3 (-2.6819, 2.3953) -> (8.9641, 2.3953)
  line L4 (8.9641, 2.3953) -> (8.9641, 0)
  line L5 (8.9641, 0) -> (0, 0)
  point P0 (11.1054, -11.3118)
  constraints: 10 end point, 4 perpendicular, 1 horizontal, 1 point on line
extrude "Extrusión21" cut sketch "Boceto27" along normal mid plane 10
sketch "Boceto28" plane through (7.5, 11.3118, 0) normal (0, 1, 0) x (1, 0, 0)
  line L0 (-3.3554, -0.5) -> (-3.7554, -0.5)
  line L1 (-3.7554, -0.5) -> (-3.7554, -0.1)
  line L2 (-3.7554, -0.1) -> (-3.3554, -0.1)
  line L3 (-3.3554, -0.1) -> (-3.3554, -0.5)
  line L4 (-3.9828, -0.7) -> (-3.0054, -0.7)
  line L5 (-3.0054, -0.7) -> (-3.0054, 0.1)
  line L6 (-3.0054, 0.1) -> (-4.0438, 0.1)
  line L7 (0.3, -3.2054) -> (0.3, -3.8054)
  line L8 (0.3, -3.8054) -> (-0.3, -3.8054)
  line L9 (-0.3, -3.8054) -> (-0.3, -3.2054)
  line L10 (-0.3, -3.2054) -> (0.3, -3.2054)
  arc A0 (0.706, -3.9817) -> (-0.706, -3.9817) centre (0, -3.6054) ccw
  line L11 (3.3554, -0.5) -> (3.3554, -0.1)
  line L12 (3.3554, -0.1) -> (3.7554, -0.1)
  line L13 (3.7554, -0.1) -> (3.7554, -0.5)
  line L14 (3.7554, -0.5) -> (3.3554, -0.5)
  line L15 (3.0054, 0.1) -> (3.0054, -0.7)
  line L16 (3.0054, -0.7) -> (3.9828, -0.7)
  line L17 (4.0438, 0.1) -> (3.0054, 0.1)
  line L18 (-3.3554, -0.1) -> (-3.7554, -0.1)
  circle A1 centre (0, -3.5054) radius 0.1
  circle A2 centre (-3.5554, -0.3) radius 0.1
  circle A3 centre (3.5554, -0.3) radius 0.1
  line L19 (4.0438, 0.1) -> (4.0438, 0)
  arc A4 (3.9828, -0.7) -> (4.0438, 0) centre (0, 0) ccw
  arc A5 (-0.706, -3.9817) -> (0.706, -3.9817) centre (0, 0) ccw
  arc A6 (-4.0438, 0) -> (-3.9828, -0.7) centre (0, 0) ccw
  line L20 (-4.0438, 0) -> (-4.0438, 0.1)
  point P0 (-7.5, 0)
  point P1 (-7.5, 0)
  dimension "d102" = 0.2
  dimension "d103" = 0.2
  dimension "d104" = 0.2
  constraints: 42 end point, 8 point on circle, 7 centre point
  measures "d102" diameter of A1
  measures "d103" diameter of A2
  measures "d104" diameter of A3
extrude "Extrusión22" add sketch "Boceto28" against normal blind 0.25 contours L0 L1 L2 L3 | A6 L20 L6 L5 L4 | L7 L8 L9 L10 | A5 A0 | L11 L12 L13 L14 | L17 L19 A4 L16 L15
sketch "Boceto29" plane through (7.5, 11.3118, 0) normal (0, 1, 0) x (1, 0, 0)
  circle A0 centre (0, -3.5054) radius 0.1 projected
  arc A1 (-3.5993, -0.2101) -> (-3.5836, -0.3959) centre (0, 0) ccw projected
  arc A2 (-3.5836, -0.3959) -> (-3.5993, -0.2101) centre (-3.5554, -0.3) ccw projected
  arc A3 (3.5836, -0.3959) -> (3.5993, -0.2101) centre (0, 0) ccw projected
  arc A4 (3.5993, -0.2101) -> (3.5836, -0.3959) centre (3.5554, -0.3) ccw projected
  arc A5 (0.7951, -3.5166) -> (-0.7951, -3.5166) centre (0, -3.6054) ccw projected
  arc A6 (-3.5368, -0.7) -> (-0.7951, -3.5166) centre (0, 0) ccw projected
  line L0 (-3.0054, -0.7) -> (-3.5368, -0.7) projected
  line L1 (-3.0054, 0.1) -> (-3.0054, -0.7) projected
  line L2 (-4.0978, 0.1) -> (-3.0054, 0.1) projected
  line L3 (-4.0978, 0) -> (-4.0978, 0.1) projected
  arc A7 (-4.0978, 0) -> (4.0978, 0) centre (0, 0) ccw projected
  line L4 (4.0978, 0.1) -> (4.0978, 0) projected
  line L5 (3.0054, 0.1) -> (4.0978, 0.1) projected
  line L6 (3.0054, -0.7) -> (3.0054, 0.1) projected
  line L7 (3.5368, -0.7) -> (3.0054, -0.7) projected
  arc A8 (0.7951, -3.5166) -> (3.5368, -0.7) centre (0, 0) ccw projected
  circle A9 centre (3.5554, -0.3) radius 0.1
  circle A10 centre (-3.5554, -0.3) radius 0.1
  point P0 (-7.5, 0)
  constraints: 2 centre point, 2 coincident
extrude "Extrusión23" cut sketch "Boceto29" against normal blind 0.25 contours A2 A1 | A1 A10 | A4 A3 | A3 A9
